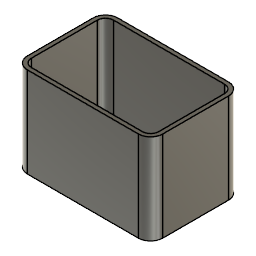
▢-150×100×4.5 (Autodesk Fusion 360 design; units mm, degrees)
Autodesk Fusion 360 part; units mm, degrees
sketch "スケッチ1" plane through (0, 0, 0) normal (0, 0, 1) x (1, 0, 0)
  line L0 (558.2333, -18.8104) -> (681.2333, -18.8104)
  line L1 (558.2333, -14.3104) -> (681.2333, -14.3104)
  line L2 (681.2333, 81.1896) -> (558.2333, 81.1896)
  line L3 (681.2333, 76.6896) -> (558.2333, 76.6896)
  arc A0 (558.2333, 81.1896) -> (544.7333, 67.6896) centre (558.2333, 67.6896) ccw
  arc A1 (558.2333, 76.6896) -> (549.2333, 67.6896) centre (558.2333, 67.6896) ccw
  arc A2 (544.7333, -5.3104) -> (558.2333, -18.8104) centre (558.2333, -5.3104) ccw
  arc A3 (549.2333, -5.3104) -> (558.2333, -14.3104) centre (558.2333, -5.3104) ccw
  line L4 (544.7333, 67.6896) -> (544.7333, -5.3104)
  line L5 (549.2333, 67.6896) -> (549.2333, -5.3104)
  arc A4 (694.7333, 67.6896) -> (681.2333, 81.1896) centre (681.2333, 67.6896) ccw
  arc A5 (690.2333, 67.6896) -> (681.2333, 76.6896) centre (681.2333, 67.6896) ccw
  arc A6 (681.2333, -18.8104) -> (694.7333, -5.3104) centre (681.2333, -5.3104) ccw
  arc A7 (681.2333, -14.3104) -> (690.2333, -5.3104) centre (681.2333, -5.3104) ccw
  line L6 (694.7333, -5.3104) -> (694.7333, 67.6896)
  line L7 (690.2333, -5.3104) -> (690.2333, 67.6896)
  point P0 (619.7333, 31.1896)
extrude "押し出し1" add sketch "スケッチ1" along normal blind 100
